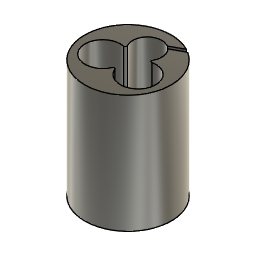
cable gland inserts v3 (Autodesk Fusion 360 design; units mm, degrees)
Autodesk Fusion 360 part; units mm, degrees
sketch "Sketch2" plane through (0, 0, 0) normal (0, 0, 1) x (1, 0, 0) in component "2x12AWG_silicone, 1x DS18B"
  circle A0 centre (0, 0) radius 5.5
  dimension "d8" = 11
  constraint coincident A0.centre origin
  measures "d8" diameter of A0
extrude "Extrude1" add sketch "Sketch2" along normal blind 15 in component "2x12AWG_silicone, 1x DS18B"
sketch "Sketch3" plane through (0, 0, 15) normal (0, 0, 1) x (-1, 0, 0) in component "2x12AWG_silicone, 1x DS18B"
  circle A0 centre (0, 0) radius 5.5
  circle A1 centre (2.25, 0.9695) radius 2.25
  circle A2 centre (-2.25, 0.9695) radius 2.25
  circle A3 centre (0, -2.4579) radius 1.85
  circle A4 centre (0, 0) radius 4.7 construction
  dimension "d11" = 4.5
  dimension "d12" = 3.7
  dimension "d13" = 0.8
  constraint equal A1 A2
  constraint tangent A1 A2
  constraint tangent A2 A3
  constraint tangent A1 A3
  constraint horizontal A1.centre A2.centre
  constraint concentric A0 A4
  constraint tangent A2 A4
  constraint tangent A1 A4
  measures "d11" diameter of A1
  measures "d12" diameter of A3
  measures "d13" distance of A0 A4
extrude "Extrude2" cut sketch "Sketch3" against normal blind 13 contours A1 | A2 | A1 A2 A3 | A3 in component "2x12AWG_silicone, 1x DS18B"
fillet "Fillet1" radius 0.2 3 edges at (-1.0152, 0.9114, 8.5) (0, -0.9695, 8.5) (1.0152, 0.9114, 8.5) in component "2x12AWG_silicone, 1x DS18B"
sketch "Sketch4" plane through (0, 0, 15) normal (0, 0, 1) x (-1, 0, 0) in component "2x12AWG_silicone, 1x DS18B"
  arc A0 (-1.6028, -1.5341) -> (-1.8148, -1.238) centre (-1.7761, -1.4342) ccw
  arc A1 (-0.1837, 1.8599) -> (-1.8148, -1.238) centre (-2.25, 0.9695) ccw
  arc A2 (-0.1837, 1.8599) -> (0.1837, 1.8599) centre (0, 1.9391) ccw
  arc A3 (1.8148, -1.238) -> (0.1837, 1.8599) centre (2.25, 0.9695) ccw
  arc A4 (1.8148, -1.238) -> (1.6028, -1.5341) centre (1.7761, -1.4342) ccw
  arc A5 (-1.6028, -1.5341) -> (1.6028, -1.5341) centre (0, -2.4579) ccw
  circle A6 centre (0, 0) radius 5.5
  line L0 (-0.9824, -4.0255) -> (-2.539, -4.8789)
  line L1 (-1.3198, -3.7543) -> (-2.9449, -4.6452)
  dimension "d18" = 0.4
  constraint coincident A5 L0.start
  constraint coincident A6 L0.end
  constraint coincident A5 L1.start
  constraint coincident A6 L1.end
  constraint parallel L0 L1
  measures "d18" distance of L0 L1
extrude "Extrude3" cut sketch "Sketch4" against normal blind 16.5 contours A5 A6 L0 L1 in component "2x12AWG_silicone, 1x DS18B"
component "2x12AWG_silicone, 1x DS18B" placed x (1, 0, 0) y (0, 1, 0) z (0, 0, 1) at (0, 0, 0)
equation "Si12AWG = 4.6 mm"
equation "DS18B20 = 3.7 mm"
equation "clearance = 0.2 mm"
equation "gland_ID_max = 12 mm"
equation "gland_ID_min = 5.65 mm"
equation "insert_D = 9 mm"
equation "insert_L = 15 mm"
equation "d8 = gland_ID_max - 1 mm"
equation "d9 = insert_L"
equation "d11 = Si12AWG - clearance / 2"
equation "d12 = DS18B20"
